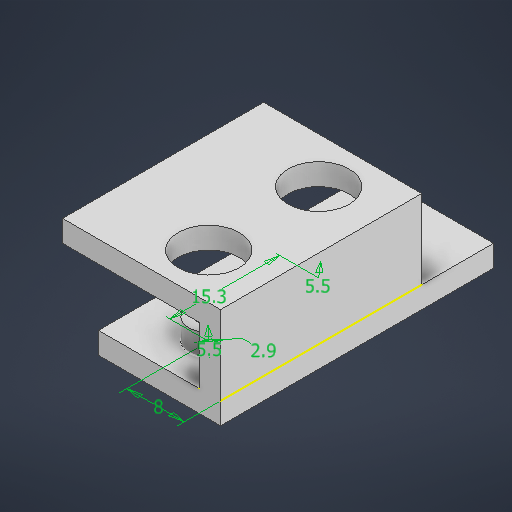
# Autodesk Inventor part: imu_housing_op
Saved by Autodesk Inventor 2025.2 (Build 292293000, 293)
## iProperties
Created: 2025-02-13
Part Number: imu_housing_op
Material: Generic
Document SubType Name: Modeling
Designer: Alex
Density: 1 g/cm^3
Appearance: Default
Author: Alex
Autodesk Inventor part; units mm, degrees
ref_plane "YZ Plane" through (0, 0, 0) normal (1, 0, 0) x (0, 1, 0)
ref_plane "XZ Plane" through (0, 0, 0) normal (0, 1, 0) x (-1, 0, 0)
ref_plane "XY Plane" through (0, 0, 0) normal (0, 0, 1) x (1, 0, 0)
sketch "Sketch1" plane through (0, 0, 0) normal (0, 0, 1) x (1, 0, 0)
  line L0 (0, 0) -> (11, 0)
  line L1 (11, 0) -> (11, 3)
  line L2 (11, 3) -> (0, 3)
  line L3 (0, 3) -> (0, 0)
  line L4 (11, 0) -> (8, 0)
  line L5 (8, 0) -> (8, 11)
  line L6 (8, 11) -> (11, 11)
  line L7 (11, 11) -> (11, 0)
  line L8 (11, 11) -> (-7, 11)
  line L9 (-7, 11) -> (-7, 14)
  line L10 (-7, 14) -> (11, 14)
  line L11 (11, 14) -> (11, 11)
  line L12 (8, 3) -> (0, 3) construction
  line L13 (4, 3) -> (4, 0) construction
  dimension "d0" = 3
  dimension "d1" = 3
  dimension "d2" = 3
  dimension "d4" = 14
  dimension "d5" = 18
  dimension "d7" = 4
  constraints: 28 end point, 6 parallel, 4 perpendicular, 3 horizontal, 3 point on line, 1 collinear, 1 midpoint
  measures "d0" distance between parallel lines of L0 L2
  measures "d1" distance between parallel lines of L7 L5
  measures "d2" distance between parallel lines of L8 L10
  measures "d4" distance between parallel lines of L0 L10
  measures "d5" distance of L9.end L10.end
  measures "d7" distance between parallel lines of L5 L13
extrude "Extrusion1" add sketch "Sketch1" along normal blind 28
sketch "Sketch2" plane through (0, 3, 0) normal (0, 1, 0) x (1, 0, 0)
  circle A0 centre (3, -6.35) radius 1.45
  circle A1 centre (3, -21.65) radius 1.45
  line L0 (8, 0) -> (8, -28) projected
  line L1 (11, 0) -> (11, -28) projected
  line L2 (11, 0) -> (11, -28) projected
  line L3 (3, -6.35) -> (3, -21.65) construction
  line L4 (3, -14) -> (8, -14) construction
  circle A2 centre (3, -21.65) radius 2.75
  circle A3 centre (3, -6.35) radius 2.75
  point P0 (0, 0)
  dimension "d10" = 8
  dimension "d11" = 2.9
  dimension "d12" = 15.3
  dimension "d13" = 5.5
  dimension "d14" = 5.5
  constraints: 4 centre point, 4 end point, 2 coincident, 2 midpoint, 1 equal radius, 1 perpendicular, 1 vertical, 1 vertical alignment
  measures "d10" distance from line of L1 L3.end
  measures "d11" diameter of A1
  measures "d12" distance of L3.start L3.end
  measures "d13" diameter of A2
  measures "d14" diameter of A3
extrude "Extrusion2" cut sketch "Sketch2" against normal up to surface (3 mm away) contours A0 | A1
extrude "Extrusion4" add sketch "Sketch2" along normal blind 3
sketch "Sketch3" plane through (-7, 14, 0) normal (0, 1, 0) x (1, 0, 0)
  circle A0 centre (10, -21.65) radius 2.75 construction
  circle A1 centre (10, -6.35) radius 2.75 construction
  circle A2 centre (10, -6.35) radius 4.25
  circle A3 centre (10, -21.65) radius 4.25
  point P0 (7, 0)
  dimension "d21" = 1.5
  dimension "d22" = 1.5
  constraints: 2 centre point
  measures "d21" radial gap between concentric circles of A1 A2
  measures "d22" radial gap between concentric circles of A0 A3
extrude "Extrusion5" cut sketch "Sketch3" against normal up to next
sketch "Sketch4" plane through (0, 0, 0) normal (-1, 0, 0) x (0, 0, 1)
  line L0 (0, 0) -> (28, 0) projected
  line L1 (28, 3) -> (28, 0) projected
  line L2 (0, 3) -> (28, 3) projected
  line L3 (0, 3) -> (0, 0) projected
extrude "Extrusion6" add sketch "Sketch4" along normal blind 6
sketch "Sketch8" plane through (-7, 11, 0) normal (-1, 0, 0) x (0, 0, 1)
  line L0 (0, 3) -> (0, 0) projected
  line L1 (0, 0) -> (28, 0) projected
  line L2 (28, 3) -> (28, 0) projected
  line L3 (0, 3) -> (28, 3) projected
  point P0 (0, -11)
extrude "Extrusion10" add sketch "Sketch8" along normal blind 4
extrude "Extrusion11" add sketch "Sketch8" along normal blind 4
sketch "Sketch10" plane through (0, 0, 0) normal (0, 0, -1) x (-1, 0, 0)
  line L0 (-11, 0) -> (6, 0) projected
  line L1 (-11, 0) -> (-11, 14) projected
  line L2 (6, 0) -> (-11, 0)
  line L3 (-11, 0) -> (-11, 3)
  line L4 (-11, 3) -> (6, 3)
  line L5 (6, 3) -> (6, 0)
  line L6 (-8, 3) -> (6, 3) projected
  point P0 (0, 0)
  constraints: 8 end point, 2 parallel, 1 collinear, 1 horizontal, 1 perpendicular, 1 point on line
extrude "Extrusion13" add sketch "Sketch10" along normal blind 10
sketch "Sketch11" plane through (-6, 0, 28) normal (0, -1, 0) x (1, 0, 0)
  circle A0 centre (9, -21.65) radius 1.45 construction
  circle A1 centre (9, -6.35) radius 1.45 construction
  line L0 (17, -38) -> (17, 0) construction
  line L1 (17, 0) -> (0, 0) construction
  line L2 (0, 0) -> (0, -38) construction
  line L3 (17, -38) -> (0, -38) construction
  circle A2 centre (8.5, -33.5) radius 2
  point P0 (6, -28)
  point P1 (8.5, -38)
  dimension "d44" = 4.5
  dimension "d45" = 4
  constraints: 1 centre point, 1 midpoint, 1 vertical alignment
  measures "d44" distance from line of A2.centre L3
  measures "d45" diameter of A2
extrude "Extrusion14" cut sketch "Sketch11" against normal up to next
equation "\"d15\" = d14"
body "Solid1"
